Autodesk Fusion 360 part; units mm, degrees
note: some values were not read from the file. Chosen so that the rebuilt part matches the saved one: which face or edge a step refers to. Set by a fixed rule: which sketch regions a step uses.
(part 2 of 2)
sketch "スケッチ43" plane through (0, 0, 2) normal (0, 0, 1) x (-1, 0, 0)
  circle A0 centre (-235, -75.5) radius 12.5
  circle A1 centre (-182, -113.5) radius 12.5
  line L0 (-160, -28.95) -> (-160, -2)
  line L1 (-160, -2) -> (-294, -2)
  line L2 (-294, -2) -> (-294, -66)
  line L3 (-294, -66) -> (-268, -66)
  line L4 (-268, -66) -> (-268, -73)
  line L5 (-268, -73) -> (-274, -73)
  line L6 (-274, -73) -> (-274, -78)
  line L7 (-274, -78) -> (-283, -78)
  line L8 (-283, -78) -> (-283, -85)
  line L9 (-283, -85) -> (-292, -85)
  line L10 (-292, -85) -> (-292, -138)
  line L11 (-292, -138) -> (-283, -138)
  line L12 (-283, -138) -> (-283, -149)
  line L13 (-283, -149) -> (-274, -149)
  line L14 (-274, -149) -> (-274, -156)
  line L15 (-274, -156) -> (-196, -156)
  line L16 (-196, -156) -> (-196, -149)
  line L17 (-196, -149) -> (-187, -149)
  line L18 (-187, -149) -> (-187, -136.5)
  line L19 (-187, -136.5) -> (-177, -136.5)
  line L20 (-177, -136.5) -> (-177, -149)
  line L21 (-177, -149) -> (-168, -149)
  line L22 (-168, -149) -> (-168, -156)
  line L23 (-168, -156) -> (-160, -156)
  line L24 (-160, -156) -> (-160, -116.7)
  line L25 (-160, -116.7) -> (-150.5, -116.7)
  line L26 (-150.5, -116.7) -> (-150.5, -106.3)
  line L27 (-150.5, -106.3) -> (-160, -106.3)
  line L28 (-160, -106.3) -> (-160, -78)
  line L29 (-160, -78) -> (-177, -78)
  line L30 (-177, -78) -> (-177, -85)
  line L31 (-177, -85) -> (-187, -85)
  line L32 (-187, -85) -> (-187, -78)
  line L33 (-187, -78) -> (-196, -78)
  line L34 (-196, -78) -> (-196, -73)
  line L35 (-196, -73) -> (-172, -73)
  line L36 (-172, -73) -> (-172, -66)
  line L37 (-172, -66) -> (-169, -66)
  line L38 (-169, -66) -> (-169, -73)
  line L39 (-169, -73) -> (-160, -73)
  line L40 (-160, -73) -> (-160, -39.35)
  line L41 (-160, -39.35) -> (-150.5, -39.35)
  line L42 (-150.5, -39.35) -> (-150.5, -28.95)
  line L43 (-150.5, -28.95) -> (-160, -28.95)
  line L44 (-172, -66) -> (-170.5, -66)
  line L45 (-170.5, -66) -> (-170.5, -30.5)
  line L46 (-170.5, -30.5) -> (-172, -30.5)
  line L47 (-172, -30.5) -> (-172, -66)
  dimension "d246" = 1.5
  dimension "d247" = 35.5
  constraint horizontal L44
  constraint vertical L45
  constraint horizontal L46
  constraint vertical L47
  constraint coincident L36.end L37.start
  measures "d246" distance of L36.end L44.end
  measures "d247" distance of L36.end L46.end
sketch "スケッチ44" plane through (0, 0, 2) normal (0, 0, 1) x (-1, 0, 0)
  circle A0 centre (-170.5, -30.5) radius 12.5
  line L0 (-170.5, -30.5) -> (-100.5, -30.5)
  line L1 (-100.5, -30.5) -> (-100.5, -13.6564)
  line L2 (-100.5, -13.6564) -> (-170.5, -13.6564)
  line L3 (-170.5, -13.6564) -> (-170.5, -30.5)
  circle A1 centre (-100.5, -30.5) radius 12.5
  point P0 (-170.5, -30.5)
  dimension "d248" = 25
  dimension "d249" = 70
  dimension "d250" = 25
  constraint coincident P0 A0.centre
  constraint horizontal L0
  constraint vertical L1
  constraint horizontal L2
  constraint vertical L3
  constraint coincident L0.end L1.start
  measures "d248" diameter of A0
  measures "d249" distance of P0 L0.end
  measures "d250" diameter of A1
extrude "押し出し75" add 1 faces at (83.6, 39.75, 1.6667) along direction (0, -1, 0) blind 16 on bodies 4 bodies 4
extrude "押し出し76" cut 1 faces at (153.6667, 39.35, 1.6667) along direction (0, -1, 0) blind 20 on bodies 1 bodies 1
extrude "押し出し77" cut sketch "スケッチ44" against normal blind 13 contours A0 L0 L3 | A0 L0 L3 | L0 L1 A1 picked at (-92.2132, -31.121) bodies 1 4
extrude "押し出し78" add 1 faces at (86.8, 117.1, 1.3333) along direction (0, -1, 0) blind 14 on bodies 4 bodies 4
extrude "押し出し79" cut 1 faces at (153.6667, 106.3, 1.6667) along direction (0, 1, 0) blind 18 on bodies 1 bodies 1
sketch "スケッチ45" plane through (0, 0, 2) normal (0, 0, 1) x (-1, 0, 0)
  line L0 (-90, -117.1) -> (-90, -156)
  line L1 (-90, -156) -> (-20, -156)
  line L2 (-20, -156) -> (-20, -149)
  line L3 (-20, -149) -> (-11, -149)
  line L4 (-11, -149) -> (-11, -138)
  line L5 (-11, -138) -> (-2, -138)
  line L6 (-2, -138) -> (-2, -85)
  line L7 (-2, -85) -> (-11, -85)
  line L8 (-11, -85) -> (-11, -78)
  line L9 (-11, -78) -> (-20, -78)
  line L10 (-20, -78) -> (-20, -73)
  line L11 (-20, -73) -> (-2, -73)
  line L12 (-2, -73) -> (-2, -2)
  line L13 (-2, -2) -> (-90, -2)
  line L14 (-90, -2) -> (-90, -23.7177)
  arc A0 (-90, -37.2823) -> (-90, -23.7177) centre (-100.5, -30.5) ccw
  line L15 (-90, -37.2823) -> (-90, -103.1)
  line L16 (-90, -103.1) -> (-90, -105.9)
  line L17 (-90, -105.9) -> (-90, -117.1)
  circle A1 centre (-59, -75.5) radius 12.5
  line L18 (-90, -2) -> (-75, -2)
  line L19 (-75, -2) -> (-75, -9.5)
  line L20 (-75, -9.5) -> (-90, -9.5)
  line L21 (-90, -9.5) -> (-90, -2)
  line L22 (-75, -2) -> (-82.5, -2)
  line L23 (-82.5, -2) -> (-82.5, -17)
  line L24 (-82.5, -17) -> (-75, -17)
  line L25 (-75, -17) -> (-75, -2)
  dimension "d261" = 7.5
  dimension "d262" = 7.5
  dimension "d263" = 15
  constraint horizontal L18
  constraint vertical L19
  constraint horizontal L20
  constraint vertical L21
  constraint coincident L13.end L14.start
  constraint horizontal L22
  constraint vertical L23
  constraint horizontal L24
  constraint vertical L25
  measures "d261" distance of L13.end L20.end
  measures "d262" distance of L18.end L22.end
  measures "d263" distance of L18.end L24.end
extrude "押し出し80" cut sketch "スケッチ45" against normal blind 12 contours L13 L14 L18 L20 L21 L23 | L13 L18 L19 L20 L22 L23 L25 | L20 L23 L24 L25 bodies 4
sketch "スケッチ46" plane through (0, 0, 2) normal (0, 0, 1) x (1, 0, 0)
  line L0 (75, 17) -> (145, 17)
  line L1 (145, 17) -> (145, 2)
  line L2 (145, 2) -> (75, 2)
  line L3 (75, 2) -> (75, 17)
  line L4 (145, 2) -> (160, 2)
  line L5 (160, 2) -> (160, 9.5)
  line L6 (160, 9.5) -> (145, 9.5)
  line L7 (145, 9.5) -> (145, 2)
  line L8 (145, 2) -> (152.5, 2)
  line L9 (152.5, 2) -> (152.5, 17)
  line L10 (152.5, 17) -> (145, 17)
  line L11 (145, 17) -> (145, 2)
  point P0 (75, 17)
  dimension "d266" = 70
  dimension "d267" = 15
  dimension "d268" = 7.5
  dimension "d269" = 7.5
  dimension "d270" = 15
  constraint horizontal L0
  constraint vertical L1
  constraint horizontal L2
  constraint vertical L3
  constraint coincident P0 L0.start
  constraint horizontal L4
  constraint vertical L5
  constraint horizontal L6
  constraint vertical L7
  constraint horizontal L8
  constraint vertical L9
  constraint horizontal L10
  constraint vertical L11
  measures "d266" distance of P0 L0.end
  measures "d267" distance of L1.end L4.end
  measures "d268" distance of L1.end L6.end
  measures "d269" distance of L1.end L8.end
  measures "d270" distance of L1.end L0.end
sketch "スケッチ47" plane through (0, 0, 2) normal (0, 0, 1) x (1, 0, 0)
  line L0 (145, 17) -> (145.15, 17)
  line L1 (145.15, 17) -> (145.15, 16.85)
  line L2 (145.15, 16.85) -> (145, 16.85)
  line L3 (145, 16.85) -> (145, 17)
  line L4 (145.15, 16.85) -> (152.35, 16.85)
  line L5 (152.35, 16.85) -> (152.35, 2.15)
  line L6 (152.35, 2.15) -> (145.15, 2.15)
  line L7 (145.15, 2.15) -> (145.15, 16.85)
  line L8 (145.15, 2.15) -> (160.5, 2.15)
  line L9 (160.5, 2.15) -> (160.5, 9.35)
  line L10 (160.5, 9.35) -> (145.15, 9.35)
  line L11 (145.15, 9.35) -> (145.15, 2.15)
  point P0 (145, 17)
  dimension "d271" = 0.15
  dimension "d272" = 0.15
  dimension "d273" = 7.2
  dimension "d274" = 14.7
  dimension "d275" = 7.2
  constraint horizontal L0
  constraint vertical L1
  constraint horizontal L2
  constraint vertical L3
  constraint coincident P0 L0.start
  constraint horizontal L4
  constraint vertical L5
  constraint horizontal L6
  constraint vertical L7
  constraint horizontal L8
  constraint vertical L9
  constraint horizontal L10
  constraint vertical L11
  measures "d271" distance of P0 L0.end
  measures "d272" distance of P0 L2.end
  measures "d273" distance of L1.end L4.end
  measures "d274" distance of L1.end L6.end
  measures "d275" distance of L6.end L10.end
extrude "押し出し81" add sketch "スケッチ47" against normal blind 1 contours L4 L5 L7 L10 | L5 L6 L7 L8 L10 L11 | L5 L8 L9 L10 bodies 1
sketch "スケッチ48" plane through (0, 0, 0) normal (0, 0, 1) x (1, 0, 0)
  line L0 (182, 113.5) -> (90, 113.5)
  line L1 (90, 113.5) -> (90, 100)
  line L2 (90, 100) -> (182, 100)
  line L3 (182, 100) -> (182, 113.5)
  line L4 (90, 37.2823) -> (90, 103.1)
  line L5 (90, 113.5) -> (75, 113.5)
  line L6 (75, 113.5) -> (75, 109.75)
  line L7 (75, 109.75) -> (90, 109.75)
  line L8 (90, 109.75) -> (90, 113.5)
  line L9 (90, 113.5) -> (75, 113.5)
  line L10 (75, 113.5) -> (75, 117.25)
  line L11 (75, 117.25) -> (90, 117.25)
  line L12 (90, 117.25) -> (90, 113.5)
  line L13 (75, 117.25) -> (82.5, 117.25)
  line L14 (82.5, 117.25) -> (82.5, 124.75)
  line L15 (82.5, 124.75) -> (75, 124.75)
  line L16 (75, 124.75) -> (75, 117.25)
  line L17 (75, 109.75) -> (82.5, 109.75)
  line L18 (82.5, 109.75) -> (82.5, 102.25)
  line L19 (82.5, 102.25) -> (75, 102.25)
  line L20 (75, 102.25) -> (75, 109.75)
  point P0 (182, 113.5)
  dimension "d278" = 15
  dimension "d279" = 3.75
  dimension "d280" = 15
  dimension "d281" = 3.75
  dimension "d282" = 7.5
  dimension "d283" = 7.5
  dimension "d284" = 7.5
  dimension "d285" = 7.5
  constraint horizontal L0
  constraint vertical L1
  constraint horizontal L2
  constraint vertical L3
  constraint coincident L1.end L4
  constraint coincident P0 L0.start
  constraint horizontal L5
  constraint vertical L6
  constraint horizontal L7
  constraint vertical L8
  constraint horizontal L9
  constraint vertical L10
  constraint horizontal L11
  constraint vertical L12
  constraint horizontal L13
  constraint vertical L14
  constraint horizontal L15
  constraint vertical L16
  constraint horizontal L17
  constraint vertical L18
  constraint horizontal L19
  constraint vertical L20
  measures "d278" distance of L0.end L5.end
  measures "d279" distance of L0.end L7.end
  measures "d280" distance of L0.end L5.end
  measures "d281" distance of L0.end L11.end
  measures "d282" distance of L10.end L13.end
  measures "d283" distance of L10.end L15.end
  measures "d284" distance of L6.end L17.end
  measures "d285" distance of L6.end L19.end
extrude "押し出し82" cut sketch "スケッチ48" along normal blind 5 contours L1 L5 L6 L7 L8 L9 L17 | L5 L9 L10 L11 L12 L13 | L7 L17 L18 L19 L20 | L11 L13 L14 L15 L16 bodies 4
sketch "スケッチ49" plane through (0, 0, 0) normal (0, 0, 1) x (1, 0, 0)
  line L0 (75, 124.75) -> (145, 124.75)
  line L1 (145, 124.75) -> (145, 102.25)
  line L2 (145, 102.25) -> (75, 102.25)
  line L3 (75, 102.25) -> (75, 124.75)
  line L4 (145, 124.75) -> (152.5, 124.75)
  line L5 (152.5, 124.75) -> (152.5, 102.25)
  line L6 (152.5, 102.25) -> (145, 102.25)
  line L7 (145, 102.25) -> (145, 124.75)
  line L8 (90, 117.25) -> (160, 117.25)
  line L9 (160, 117.25) -> (160, 109.75)
  line L10 (160, 109.75) -> (90, 109.75)
  line L11 (90, 109.75) -> (90, 117.25)
  line L12 (145, 124.75) -> (145.15, 124.75)
  line L13 (145.15, 124.75) -> (145.15, 124.6)
  line L14 (145.15, 124.6) -> (145, 124.6)
  line L15 (145, 124.6) -> (145, 124.75)
  line L16 (145.15, 124.6) -> (152.35, 124.6)
  line L17 (152.35, 124.6) -> (152.35, 102.4)
  line L18 (152.35, 102.4) -> (145.15, 102.4)
  line L19 (145.15, 102.4) -> (145.15, 124.6)
  line L20 (160, 117.25) -> (159.85, 117.25)
  line L21 (159.85, 117.25) -> (159.85, 117.1)
  line L22 (159.85, 117.1) -> (160, 117.1)
  line L23 (160, 117.1) -> (160, 117.25)
  line L24 (159.85, 117.1) -> (145.15, 117.1)
  line L25 (145.15, 117.1) -> (145.15, 109.9)
  line L26 (145.15, 109.9) -> (159.85, 109.9)
  line L27 (159.85, 109.9) -> (159.85, 117.1)
  point P0 (75, 124.75)
  point P1 (90, 117.25)
  dimension "d288" = 70
  dimension "d289" = 22.5
  dimension "d290" = 7.5
  dimension "d291" = 22.5
  dimension "d292" = 70
  dimension "d293" = 7.5
  dimension "d294" = 0.15
  dimension "d295" = 0.15
  dimension "d296" = 7.2
  dimension "d297" = 22.2
  dimension "d298" = 0.15
  dimension "d299" = 0.15
  dimension "d300" = 14.7
  dimension "d301" = 7.2
  constraint horizontal L0
  constraint vertical L1
  constraint horizontal L2
  constraint vertical L3
  constraint coincident P0 L0.start
  constraint horizontal L4
  constraint vertical L5
  constraint horizontal L6
  constraint vertical L7
  constraint horizontal L8
  constraint vertical L9
  constraint horizontal L10
  constraint vertical L11
  constraint coincident P1 L8.start
  constraint horizontal L12
  constraint vertical L13
  constraint horizontal L14
  constraint vertical L15
  constraint horizontal L16
  constraint vertical L17
  constraint horizontal L18
  constraint vertical L19
  constraint horizontal L20
  constraint vertical L21
  constraint horizontal L22
  constraint vertical L23
  constraint horizontal L24
  constraint vertical L25
  constraint horizontal L26
  constraint vertical L27
  measures "d288" distance of P0 L0.end
  measures "d289" distance of P0 L2.end
  measures "d290" distance of L0.end L4.end
  measures "d291" distance of L0.end L1.end
  measures "d292" distance of P1 L8.end
  measures "d293" distance of P1 L10.end
  measures "d294" distance of L0.end L12.end
  measures "d295" distance of L0.end L14.end
  measures "d296" distance of L13.end L16.end
  measures "d297" distance of L13.end L18.end
  measures "d298" distance of L8.end L20.end
  measures "d299" distance of L8.end L22.end
  measures "d300" distance of L21.end L24.end
  measures "d301" distance of L21.end L26.end
extrude "押し出し83" add sketch "スケッチ49" along normal blind 2 separate body contours L8 L16 L17 L19 | L10 L17 L18 L19 | L17 L19 L24 L25 L26 | L5 L24 L26 L27 makes body 6 at (147.55, 112.3, 0) makes body 7 at (147.55, 107.3, 0) makes body 8 at (147.55, 122.15, 0) makes body 9 at (154.95, 114.7, 0)
extrude "押し出し84" add 1 faces at (147.55, 117.25, 0.6667) along direction (0, -1, 0) blind 10 on bodies 8 bodies 6 8 7
extrude "押し出し85" cut 2 faces at (154.95, 114.7, 0) (147.55, 109.8, 0) along direction (0, 0, 1) blind 1 on bodies 6 9 bodies 6 9
extrude "押し出し86" add 1 faces at (159.85, 112.3, 1.3333) along direction (1, 0, 0) blind 0.5 on bodies 9 bodies 1 9
extrude "押し出し87" add 1 faces at (152.5, 114.7, 1.3333) along direction (-1, 0, 0) blind 1 on bodies 1 bodies 1 6
extrude "押し出し88" add sketch "スケッチ34" along normal blind 5 bodies 1
extrude "押し出し89" cut 1 faces at (274.3333, 73, 28) along direction (0, 1, 0) blind 15 on bodies 1 bodies 1
extrude "押し出し90" add 1 faces at (5, 85, 11.6667) along direction (0, 1, 0) blind 10 on bodies 4 bodies 4
extrude "押し出し91" add 1 faces at (5, 138, 21.3333) along direction (0, -1, 0) blind 6 on bodies 4 bodies 4
extrude "押し出し92" cut 1 faces at (5, 132, 21.3333) along direction (0, 1, 0) blind 5 on bodies 4 bodies 4
extrude "押し出し93" cut 1 faces at (5, 95, 11.6667) along direction (0, -1, 0) blind 5 on bodies 4 bodies 4
extrude "押し出し94" add 1 faces at (168, 151.3333, 21) along direction (-1, 0, 0) blind 3 on bodies 1 bodies 1
extrude "押し出し95" add 1 faces at (20, 151.3333, 21) along direction (1, 0, 0) blind 3 on bodies 4 bodies 4
extrude "押し出し96" add 1 faces at (196, 151.3333, 21) along direction (1, 0, 0) blind 3 on bodies 1 bodies 1
extrude "押し出し97" add 1 faces at (274, 151.3333, 21) along direction (-1, 0, 0) blind 3 on bodies 1 bodies 1
extrude "押し出し98" add 1 faces at (289, 138, 21.3333) along direction (0, -1, 0) blind 1 on bodies 1 bodies 1
extrude "押し出し99" add 1 faces at (289, 85, 21.3333) along direction (0, 1, 0) blind 3 on bodies 1 bodies 1
extrude "押し出し100" add 1 faces at (20, 76.3333, 9.3333) along direction (1, 0, 0) blind 3 on bodies 4 bodies 4
extrude "押し出し101" add 1 faces at (196, 74.6667, 9.3333) along direction (1, 0, 0) blind 3 on bodies 1 bodies 1
extrude "押し出し102" add 2 faces at (204.6667, 0, 21) (30, 0, 11) along direction (0, -1, 0) blind 2 on bodies 1 4 bodies 1 4
extrude "押し出し103" cut 2 faces at (55.6667, 2, 21.3333) (207, 2, 21.3333) along direction (0, -1, 0) blind 2 on bodies 1 4 bodies 1 4
sketch "スケッチ50" plane through (75, 0, 0) normal (1, 0, 0) x (0, 1, 0)
  line L0 (0, 1) -> (17, 1)
  line L1 (17, 1) -> (17, 2)
  line L2 (17, 2) -> (0, 2)
  line L3 (0, 2) -> (0, 1)
  line L4 (0, 1) -> (2, 1)
  line L5 (2, 1) -> (2, 2)
  line L6 (2, 2) -> (0, 2)
  line L7 (0, 2) -> (0, 1)
  dimension "d344" = 2
  constraint horizontal L4
  constraint vertical L5
  constraint horizontal L6
  constraint vertical L7
  constraint coincident L0.start L3.end
  measures "d344" distance of L0.start L4.end
extrude "押し出し104" add sketch "スケッチ50" along normal blind 15 contours L0 L2 L3 L4 L5 L6 L7 bodies 4
extrude "押し出し105" add 3 faces at (14, 73, 9.3333) (163, 73, 9.3333) (190, 73, 16.6667) along direction (0, -1, 0) blind 2 on bodies 1 4 bodies 4 1
extrude "押し出し106" add 1 faces at (170, 66, 9.3333) along direction (0, -1, 0) blind 1 on bodies 1 bodies 1
extrude "押し出し107" add 1 faces at (183.6667, 136.5, 11.6667) along direction (0, -1, 0) blind 2 on bodies 1 bodies 1
sketch "スケッチ7" plane through (0, 0, 2) normal (0, 0, 1) x (-1, 0, 0)
  line L0 (-222, -2) -> (-97, -2)
  line L1 (-97, -2) -> (-97, -66)
  line L2 (-97, -66) -> (-222, -66)
  line L3 (-222, -66) -> (-222, -2)
  point P0 (-222, -2)
  dimension "d19" = 125
  dimension "d20" = 64
  constraint horizontal L0
  constraint vertical L1
  constraint horizontal L2
  constraint vertical L3
  constraint coincident P0 L0.start
  measures "d19" distance of P0 L0.end
  measures "d20" distance of P0 L2.end
sketch "スケッチ8" plane through (0, 0, 2) normal (0, 0, 1) x (-1, 0, 0)
  line L0 (-2, -2) -> (-92, -2)
  line L1 (-92, -2) -> (-92, -60)
  line L2 (-92, -60) -> (-2, -60)
  line L3 (-2, -60) -> (-2, -2)
  point P0 (-2, -2)
  dimension "d21" = 90
  dimension "d22" = 58
  constraint horizontal L0
  constraint vertical L1
  constraint horizontal L2
  constraint vertical L3
  constraint coincident P0 L0.start
  measures "d21" distance of P0 L0.end
  measures "d22" distance of P0 L2.end
sketch "スケッチ9" plane through (0, 0, 2) normal (0, 0, 1) x (-1, 0, 0)
  line L0 (-2, -2) -> (-92, -2)
  line L1 (-92, -2) -> (-92, -57)
  line L2 (-92, -57) -> (-2, -57)
  line L3 (-2, -57) -> (-2, -2)
  line L4 (-92, -2) -> (-92, -60)
  point P0 (-2, -2)
  dimension "d23" = 55
  constraint horizontal L0
  constraint vertical L1
  constraint horizontal L2
  constraint vertical L3
  constraint coincident L1.end L4
  constraint coincident P0 L0.start
  measures "d23" distance of P0 L2.end
sketch "スケッチ10" plane through (0, 0, 2) normal (0, 0, 1) x (-1, 0, 0)
  line L0 (-76.5, -156) -> (-147.5, -156)
  line L1 (-147.5, -156) -> (-147.5, -60)
  line L2 (-147.5, -60) -> (-76.5, -60)
  line L3 (-76.5, -60) -> (-76.5, -156)
  line L4 (-147.5, -156) -> (-147.5, -60)
  point P0 (-76.5, -156)
  dimension "d24" = 96
  constraint horizontal L0
  constraint vertical L1
  constraint horizontal L2
  constraint vertical L3
  constraint coincident L1.end L4
  constraint coincident P0 L0.start
  measures "d24" distance of P0 L2.end
extrude "押し出し3" [suppressed]
extrude "押し出し4" [suppressed]
extrude "押し出し5" [suppressed]
sketch "スケッチ11" plane through (0, 0, 2) normal (0, 0, 1) x (1, 0, 0)
sketch "スケッチ12" plane through (0, 0, 2) normal (0, 0, 1) x (-1, 0, 0)
sketch "スケッチ13" plane through (0, 0, 30) normal (0, 0, 1) x (-1, 0, 0)
  line L0 (-222, -2) -> (-2, -2)
  line L1 (-2, -2) -> (-2, -156)
  line L2 (-2, -156) -> (-222, -156)
  line L3 (-222, -156) -> (-222, -2)
  line L4 (0, -158) -> (0, 0)
  line L5 (0, 0) -> (-224, 0)
  line L6 (-224, 0) -> (-224, -158)
  line L7 (-224, -158) -> (0, -158)
  line L8 (-222, 0) -> (-97, 0)
  line L9 (-97, 0) -> (-97, -64)
  line L10 (-97, -64) -> (-222, -64)
  line L11 (-222, -64) -> (-222, 0)
  dimension "d31" = 125
  dimension "d32" = 64
  constraint horizontal L8
  constraint vertical L9
  constraint horizontal L10
  constraint vertical L11
  constraint coincident L5 L8.start
  measures "d31" distance of L8.start L8.end
  measures "d32" distance of L8.start L10.end
extrude "押し出し6" [suppressed]
extrude "押し出し7" [suppressed]
extrude "押し出し8" [suppressed]
extrude "押し出し9" [suppressed]
